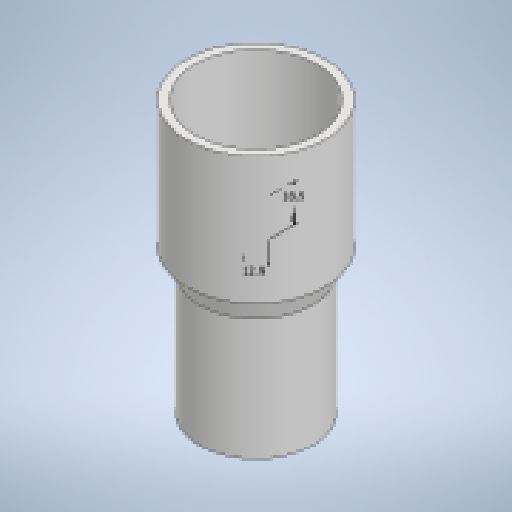
# Autodesk Inventor part: outercase
Saved by Autodesk Inventor 2025 (Build 290162000, 162)
## iProperties
Created: 2025-08-17
Part Number: outercase
Material: 一般
Document SubType Name: Modeling
Designer: gavin
Density: 1 g/cm^3
Appearance: 預設
Author: gavin
Autodesk Inventor part; units mm, degrees
ref_plane "YZ Plane" through (0, 0, 0) normal (1, 0, 0) x (0, 1, 0)
ref_plane "XZ Plane" through (0, 0, 0) normal (0, 1, 0) x (-1, 0, 0)
ref_plane "XY Plane" through (0, 0, 0) normal (0, 0, 1) x (1, 0, 0)
sketch "草圖1" plane through (0, 0, 0) normal (1, 0, 0) x (0, 1, 0)
  line L0 (0, -28.5) -> (61, -28.5)
  line L1 (61, -28.5) -> (72, -34.8304)
  line L2 (72, -34.8304) -> (136, -34.8304)
  line L3 (136, -30.6704) -> (73.1116, -30.6704)
  line L4 (73.1116, -30.6704) -> (62.1116, -24.34)
  line L5 (62.1116, -24.34) -> (0, -24.34)
  line L6 (136, -34.8304) -> (136, -30.6704)
  line L7 (0, -28.5) -> (0, -24.34)
  line L8 (-27.2, 0) -> (163.2, 0) projected
  point P0 (0, 0)
  dimension "d1" = 61
  dimension "d4" = 64
  dimension "d5" = 28.5
  dimension "d6" = 11
  dimension "d7" = 4.16
  constraints: 16 end point, 3 parallel, 1 horizontal, 1 vertical, 1 vertical alignment, 2 other
  measures "d1" distance of L0.start L0.end
  measures "d4" distance of L1.end L2.end
  measures "d5" distance from line of point (0, 0) L0
  measures "d6" horizontal distance of L0.end L1.end
  measures "d7" distance between parallel lines of L2 L3
revolve "迴轉1" add sketch "草圖1" angle 360 about axis through (0, -10, 0) along (0, 1, 0)
sketch "草圖2" plane through (0, 0, 0) normal (1, 0, 0) x (0, 1, 0)
  line L0 (72, -34.8304) -> (72, 34.8304) projected
  line L1 (72, 6.45) -> (90.9, 6.45)
  line L2 (90.9, 6.45) -> (90.9, -6.45)
  line L3 (90.9, -6.45) -> (72, -6.45)
  line L4 (72, -6.45) -> (72, 6.45)
  point P0 (0, 0)
  point P1 (72, 0)
  dimension "d9" = 18.9
  dimension "d10" = 12.9
  constraints: 8 end point, 2 midpoint, 2 parallel, 1 horizontal, 1 perpendicular
  measures "d9" distance of L2.end L3.end
  measures "d10" distance of L3.end L1.start
extrude "擠出1" cut sketch "草圖2" along normal through all
